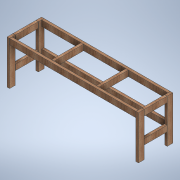
# Autodesk Inventor part: Frame Primary
Saved by Autodesk Inventor 2020.2 (Build 242310000, 310)
## iProperties
Created: 2019-12-30
Part Number: Frame Primary
Material: Wood (Birch - Stained)
Document SubType Name: Modeling
Designer: Andrew
Density: 0.1 g/cm^3
Appearance: Birch - Stained
Author: Andrew
Autodesk Inventor part; units mm, degrees
ref_plane "YZ Plane" through (0, 0, 0) normal (1, 0, 0) x (0, 1, 0)
ref_plane "XY Plane" through (0, 0, 0) normal (0, 0, 1) x (1, 0, 0)
derived "Desk Top Primary.ipt"
sketch "Primary Top" plane through (0, 0, 0) normal (0, 1, 0) x (-1, 0, 0)
  line L0 (-2713.228, 0) -> (-579.628, 0)
  line L1 (-579.628, 0) -> (-579.628, 143.3195)
  line L2 (-579.628, 143.3195) -> (-2713.228, 143.3195)
  line L3 (-2713.228, 143.3195) -> (-2713.228, 0)
  line L4 (-2713.228, 144.907) -> (-579.628, 144.907)
  line L5 (-579.628, 144.907) -> (-579.628, 288.2265)
  line L6 (-579.628, 288.2265) -> (-2713.228, 288.2265)
  line L7 (-2713.228, 288.2265) -> (-2713.228, 144.907)
  line L8 (-2713.228, 289.814) -> (-579.628, 289.814)
  line L9 (-579.628, 289.814) -> (-579.628, 433.1335)
  line L10 (-579.628, 433.1335) -> (-2713.228, 433.1335)
  line L11 (-2713.228, 433.1335) -> (-2713.228, 289.814)
  line L12 (-2713.228, 434.721) -> (-579.628, 434.721)
  line L13 (-579.628, 434.721) -> (-579.628, 578.0405)
  line L14 (-579.628, 578.0405) -> (-2713.228, 578.0405)
  line L15 (-2713.228, 578.0405) -> (-2713.228, 434.721)
  point P0 (0, 0)
sketch "Frame Primary" plane through (0, 0, 0) normal (0, 1, 0) x (-1, 0, 0)
  line L0 (-633.6121, 565.3405) -> (-2659.2439, 565.3405)
  line L1 (-2659.2439, 565.3405) -> (-2659.2439, 525.6439)
  line L2 (-2659.2439, 525.6439) -> (-633.6121, 525.6439)
  line L3 (-633.6121, 525.6439) -> (-633.6121, 565.3405)
  line L4 (-2660.8314, 565.3405) -> (-2700.528, 565.3405)
  line L5 (-2700.528, 565.3405) -> (-2700.528, 474.2815)
  line L6 (-2700.528, 474.2815) -> (-2660.8314, 474.2815)
  line L7 (-2660.8314, 474.2815) -> (-2660.8314, 565.3405)
  line L8 (-2660.8314, 472.694) -> (-2700.528, 472.694)
  line L9 (-2700.528, 472.694) -> (-2700.528, 105.3465)
  line L10 (-2700.528, 105.3465) -> (-2660.8314, 105.3465)
  line L11 (-2660.8314, 105.3465) -> (-2660.8314, 472.694)
  line L12 (-2660.8314, 103.759) -> (-2700.528, 103.759)
  line L13 (-2700.528, 103.759) -> (-2700.528, 12.7)
  line L14 (-2700.528, 12.7) -> (-2660.8314, 12.7)
  line L15 (-2660.8314, 12.7) -> (-2660.8314, 103.759)
  line L16 (-2659.2439, 12.7) -> (-633.6121, 12.7)
  line L17 (-633.6121, 12.7) -> (-633.6121, 52.3966)
  line L18 (-633.6121, 52.3966) -> (-2659.2439, 52.3966)
  line L19 (-2659.2439, 52.3966) -> (-2659.2439, 12.7)
  line L20 (-592.328, 565.3405) -> (-632.0246, 565.3405)
  line L21 (-632.0246, 565.3405) -> (-632.0246, 474.2815)
  line L22 (-632.0246, 474.2815) -> (-592.328, 474.2815)
  line L23 (-592.328, 474.2815) -> (-592.328, 565.3405)
  line L24 (-592.328, 472.694) -> (-632.0246, 472.694)
  line L25 (-632.0246, 472.694) -> (-632.0246, 105.3465)
  line L26 (-632.0246, 105.3465) -> (-592.328, 105.3465)
  line L27 (-592.328, 105.3465) -> (-592.328, 472.694)
  line L28 (-592.328, 12.7) -> (-632.0246, 12.7)
  line L29 (-632.0246, 12.7) -> (-632.0246, 103.759)
  line L30 (-632.0246, 103.759) -> (-592.328, 103.759)
  line L31 (-592.328, 103.759) -> (-592.328, 12.7)
  line L32 (-1267.0246, 53.9841) -> (-1306.7211, 53.9841)
  line L33 (-1306.7211, 53.9841) -> (-1306.7211, 524.0564)
  line L34 (-1306.7211, 524.0564) -> (-1267.0246, 524.0564)
  line L35 (-1267.0246, 524.0564) -> (-1267.0246, 53.9841)
  line L36 (-1986.1349, 53.9841) -> (-2025.8314, 53.9841)
  line L37 (-2025.8314, 53.9841) -> (-2025.8314, 524.0564)
  line L38 (-2025.8314, 524.0564) -> (-1986.1349, 524.0564)
  line L39 (-1986.1349, 524.0564) -> (-1986.1349, 53.9841)
  point P0 (0, 0)
  point P1 (-2713.228, 0)
  point P2 (-579.628, 578.0405)
  dimension "d1" = 39.6966
  dimension "d2" = 39.6966
  dimension "d3" = 39.6966
  dimension "d4" = 1.5875
  dimension "d5" = 1.5875
  dimension "d6" = 1.5875
  dimension "d7" = 1.5875
  dimension "d8" = 12.7
  dimension "d9" = 12.7
  dimension "d10" = 91.059
  dimension "d11" = 91.059
  dimension "d12" = 12.7
  dimension "d13" = 39.6966
  dimension "d14" = 91.059
  dimension "d15" = 91.059
  dimension "d16" = 1.5875
  dimension "d17" = 12.7
  dimension "d23" = 39.6966
  dimension "d24" = 39.6966
  dimension "d25" = 1.5875
  dimension "d26" = 1.5875
  dimension "d27" = 635
  dimension "d28" = 635
  dimension "d29" = 679.4137
  constraints: 80 end point, 20 parallel, 15 point on line, 10 horizontal, 10 perpendicular, 2 collinear
  measures "d1" distance of L2.end L0.start
  measures "d2" distance of L16.end L17.end
  measures "d3" distance of L13.end L14.end
  measures "d4" distance between parallel lines of L8 L6
  measures "d5" distance between parallel lines of L12 L10
  measures "d6" distance between parallel lines of L15 L19
  measures "d7" distance between parallel lines of L7 L1
  measures "d8" horizontal distance of point (-2713.228, 0) L13.end
  measures "d9" horizontal distance of L13.end point (-2713.228, 0)
  measures "d10" distance of L4.end L5.end
  measures "d11" distance of L12.end L13.end
  measures "d12" vertical distance of point (-579.628, 578.041) L4.end
  measures "d13" distance of L28.start L28.end
  measures "d14" distance of L22.end L20.start
  measures "d15" distance of L30.end L28.start
  measures "d16" distance between parallel lines of L17 L29
  measures "d17" horizontal distance of L20.start point (-579.628, 578.041)
  measures "d23" distance of L36.start L36.end
  measures "d24" distance of L32.start L32.end
  measures "d25" distance between parallel lines of L18 L32
  measures "d26" distance between parallel lines of L2 L34
  measures "d27" distance between parallel lines of L25 L35
  measures "d28" distance between parallel lines of L11 L37
  measures "d29" distance between parallel lines of L39 L33
extrude "Extrusion1" add sketch "Frame Primary" against normal blind 91.059 contours L3 L2 L1 L0 | L11 L10 L9 L8 | L19 L18 L17 L16 | L27 L26 L25 L24 | L32 L33 L34 L35 | L36 L37 L38 L39
derived "Desk Drawer.ipt"
extrude "Extrusion2" add sketch "Frame Primary" against normal blind 698.5 contours L7 L6 L5 L4 | L15 L14 L13 L12 | L23 L22 L21 L20 | L28 L29 L30 L31
ref_plane "Support Plane" through (0, -495.3, 0) normal (0, 1, 0) x (-1, 0, 0)
extrude "Extrusion3" add sketch "Frame Primary" along normal blind 91.059 from surface at -495.3 contours L11 L10 L9 L8 | L19 L18 L17 L16 | L27 L26 L25 L24
equation "\"d1\" = h_2x4"
equation "\"d2\" = h_2x4"
equation "\"d3\" = h_2x4"
equation "\"d4\" = plank_tol"
equation "\"d5\" = plank_tol"
equation "\"d6\" = plank_tol"
equation "\"d7\" = plank_tol"
equation "\"d9\" = d8"
equation "\"d10\" = w_2x4"
equation "\"d11\" = w_2x4"
equation "\"d12\" = d8"
equation "\"d13\" = h_2x4"
equation "\"d14\" = w_2x4"
equation "\"d15\" = w_2x4"
equation "\"d16\" = plank_tol"
equation "\"d17\" = d8"
equation "\"d23\" = h_2x4"
equation "\"d24\" = h_2x4"
equation "\"d25\" = plank_tol"
equation "\"d26\" = plank_tol"
equation "\"d18\" = w_2x4"
equation "\"d21\" = drawer_height"
equation "\"d31\" = w_2x4"
equation "\"h_2x4\" = 39.696571"
equation "\"plank_tol\" = 1.5875"
equation "\"w_2x4\" = 91.059"
equation "\"drawer_height\" = 698.5"
body "Solid1"
